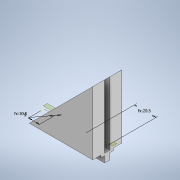
# Autodesk Inventor part: PCB_Mount_Triangle
Saved by Autodesk Inventor 2022 (Build 260153000, 153)
## iProperties
Created: 2024-03-14
Part Number: PCB_Mount_Triangle
Material: Generic
Document SubType Name: Modeling
Designer: Gotham City
Density: 1 g/cm^3
Appearance: Default
Author: Gotham City
Autodesk Inventor part; units mm, degrees
ref_plane "YZ Plane" through (0, 0, 0) normal (1, 0, 0) x (0, 1, 0)
ref_plane "XZ Plane" through (0, 0, 0) normal (0, 1, 0) x (-1, 0, 0)
ref_plane "XY Plane" through (0, 0, 0) normal (0, 0, 1) x (1, 0, 0)
sketch "Sketch1" plane through (0, 0, 0) normal (0, 0, 1) x (1, 0, 0)
  line L0 (0, 60) -> (-60, 0)
  line L1 (-60, 0) -> (0, 0)
  line L2 (0, 0) -> (0, 60)
  dimension "d0" = 45
  dimension "d1" = 60
  constraints: 6 end point, 1 horizontal, 1 perpendicular
  measures "d0" angle of L1 L0
  measures "d1" distance of L1.end L0.start
extrude "Extrusion1" add sketch "Sketch1" along normal mid plane 27.5
sketch "Sketch2" plane through (-60, 0, 13.75) normal (0, -1, 0) x (1, 0, 0)
  line L0 (0, 0) -> (0, -27.5) projected
  line L1 (60, -27.5) -> (60, 0) projected
  line L2 (0, -7.75) -> (60, -7.75)
  line L3 (60, -7.75) -> (60, -19.75)
  line L4 (60, -19.75) -> (0, -19.75)
  line L5 (0, -19.75) -> (0, -7.75)
  line L6 (30, -7.75) -> (30, 0) construction
  line L7 (0, 0) -> (60, 0) construction
  line L8 (0, -27.5) -> (60, -27.5) construction
  line L9 (30, -27.5) -> (30, -19.75) construction
  point P0 (60, -13.75)
  point P1 (0, -19.75)
  dimension "d4" = 12
  constraints: 12 end point, 4 midpoint, 2 parallel, 2 point on line, 1 collinear, 1 horizontal, 1 perpendicular
  measures "d4" distance between parallel lines of L4 L2
extrude "Extrusion2" add sketch "Sketch2" along normal blind 2.2
sketch "Sketch3" plane through (-60, -2.2, 13.75) normal (0, -1, 0) x (1, 0, 0)
  line L0 (0, -7.75) -> (0, -19.75) projected
  line L1 (60, -27.5) -> (60, 0) projected
  line L2 (0, -11.25) -> (60, -11.25)
  line L3 (60, -11.25) -> (60, -16.25)
  line L4 (60, -16.25) -> (0, -16.25)
  line L5 (0, -16.25) -> (0, -11.25)
  line L6 (30, -11.25) -> (30, -7.75) construction
  line L7 (0, -19.75) -> (60, -19.75) construction
  line L8 (30, -19.75) -> (30, -16.25) construction
  line L9 (60, -7.75) -> (0, -7.75) construction
  point P0 (60, -13.75)
  point P1 (0, -16.25)
  dimension "d7" = 5
  constraints: 12 end point, 4 midpoint, 2 parallel, 2 point on line, 1 collinear, 1 horizontal, 1 perpendicular, 1 vertical
  measures "d7" distance between parallel lines of L4 L2
extrude "Extrusion3" add sketch "Sketch3" along normal blind 6
ref_plane "Work Plane2" through (-60, 4.8, 13.75) normal (0, -1, 0) x (1, 0, 0)
sketch "Sketch4" plane through (-60, 4.8, 13.75) normal (0, -1, 0) x (1, 0, 0)
  circle A0 centre (10.5, -13.75) radius 4.5
  circle A1 centre (39.5, -13.75) radius 4.5
  line L0 (10.5, -13.75) -> (0, -13.75) construction
  line L1 (60, -16.25) -> (0, -16.25) construction
  line L2 (39.5, -13.75) -> (10.5, -13.75) construction
  line L3 (60, -11.25) -> (0, -11.25) construction
  line L4 (39.5, -13.75) -> (60, -13.75) construction
  line L5 (0, -11.25) -> (0, -16.25) construction
  dimension "d12" = 9
  dimension "d14" = 10.5
  dimension "d30" = 20.5
  constraints: 6 end point, 2 centre point, 2 parallel, 1 equal radius, 1 horizontal, 1 midpoint
  measures "d12" diameter of A0
  measures "d14" distance from line of L5 L0.start
  measures "d30" distance of L2.start L4.end
hole "Hole1" at (-49.5, 4.8, 0) at (-20.5, 4.8, 0) direction (0, -1, 0) diameter 5.5 end through all start extended yes counterbore diameter 10 counterbore depth 0.1 clearance for "Socket Head Cap Screw ISO 4762" size "M5" standard "ISO"
sketch "Sketch5" plane through (-21.6456, -2.2, -2.5) normal (0, 0, -1) x (-1, 0, 0)
  line L0 (38.3544, 0) -> (-21.6456, 0) projected
  line L1 (23.3544, 0) -> (33.3544, 0)
  line L2 (33.3544, 0) -> (33.3544, -6)
  line L3 (33.3544, -6) -> (23.3544, -6)
  line L4 (23.3544, -6) -> (23.3544, 0)
  line L5 (3.3544, 0) -> (-5.6456, 0)
  line L6 (-5.6456, 0) -> (-5.6456, -6)
  line L7 (-5.6456, -6) -> (3.3544, -6)
  line L8 (3.3544, -6) -> (3.3544, 0)
  line L9 (0, -6) -> (26.7087, -6) construction
  line L10 (-21.6456, 7) -> (38.3544, 7) construction
  line L11 (23.3544, 7) -> (32.3544, 7) projected
  point P0 (33.3544, 7)
  point P1 (42.3544, 7)
  point P2 (-5.6456, 7)
  point P3 (3.3544, 7)
  constraints: 16 end point, 4 parallel, 4 vertical alignment, 3 point on line, 2 horizontal, 2 perpendicular, 1 horizontal alignment
extrude "Extrusion5" cut sketch "Sketch5" along normal through all both and the other way through all
sketch "Sketch6" plane through (0, 0, 13.75) normal (1, 0, 0) x (0, 0, -1)
  line L0 (27.5, 60) -> (0, 60) projected
  line L1 (7.75, 0) -> (0, 0) projected
  line L2 (16.25, 60) -> (11.25, 60)
  line L3 (11.25, 60) -> (11.25, 0)
  line L4 (11.25, 0) -> (16.25, 0)
  line L5 (16.25, 0) -> (16.25, 60)
  line L6 (16.25, 30) -> (27.5, 30) construction
  line L7 (0, 0) -> (0, 60) construction
  line L8 (0, 30) -> (11.25, 30) construction
  line L9 (27.5, 60) -> (27.5, 0) construction
  point P0 (13.75, 0)
  dimension "d27" = 5
  constraints: 12 end point, 4 midpoint, 2 horizontal, 2 parallel, 2 point on line, 1 collinear, 1 perpendicular
  measures "d27" distance between parallel lines of L5 L3
extrude "Extrusion6" cut sketch "Sketch6" against normal blind 10
sketch "Sketch7" plane through (-25, -2.2, -2.5) normal (0, 0, -1) x (-1, 0, 0)
  line L0 (35, -6) -> (30, -6) projected
  line L1 (30, 0) -> (30, -6) projected
  line L2 (35, -6) -> (30, -6)
  line L3 (30, -6) -> (30, 0)
  line L4 (30, 0) -> (35, 0)
  line L5 (35, 0) -> (35, -6)
  line L6 (35, 0) -> (-25, 0) projected
  line L7 (20, 0) -> (14, -6)
  line L8 (20, -6) -> (0, -6) projected
  line L9 (20, -6) -> (20, 0) projected
  line L10 (14, -6) -> (20, -6)
  line L11 (20, -6) -> (20, 0)
  line L12 (-9, 0) -> (-9, -6) projected
  line L13 (-9, -6.0008) -> (-9, 0)
  line L14 (-9, 0) -> (-15, -6)
  line L15 (-25, -6) -> (-9, -6) projected
  line L16 (-15, -6) -> (-9, -6)
  point P0 (-25, 2.2)
  dimension "d40" = 45
  dimension "d41" = 45
  constraints: 20 end point, 4 point on line, 3 horizontal, 2 parallel, 2 perpendicular, 1 collinear
  measures "d40" angle of L9 L7
  measures "d41" angle of L14 L13
extrude "Extrusion7" cut sketch "Sketch7" against normal through all
sketch "Sketch8" plane through (0, 0, 2.5) normal (0, 0, -1) x (-1, 0, 0)
  line L0 (0, 0) -> (0, 60) projected
  line L1 (10, 50) -> (10, 0) projected
  line L2 (0, 20) -> (10, 20)
  line L3 (10, 20) -> (10, 40)
  line L4 (10, 40) -> (0, 40)
  line L5 (0, 40) -> (0, 20)
  line L6 (6, 20) -> (6, 40)
  point P0 (10, 20)
  dimension "d45" = 20
  dimension "d46" = 20
  dimension "d47" = 4
  constraints: 10 end point, 4 point on line, 2 parallel, 2 perpendicular, 1 horizontal
  measures "d45" distance from line of L0.start L2
  measures "d46" distance between parallel lines of L2 L4
  measures "d47" distance between parallel lines of L6 L1
extrude "Extrusion8" add sketch "Sketch8" along normal up to surface (5 mm away) contours L6 L4 L1 L2
chamfer "Chamfer4" distance 4 angle 45 1 edges at (-6, 40, 0)
thicken "Thicken1" operation add thickness 0.1 both sides no extend neighbours yes toward (0, 0, -1) faces at (-2, 32, -2.5)
thicken "Thicken2" operation add thickness 0.1 both sides no extend neighbours yes toward (0, 0, 1) faces at (-2, 32, 2.5)
thicken "Thicken3" operation add thickness 0.1 both sides no extend neighbours yes toward (0, 1, 0) faces at (-8.6667, 20, -0.8667) (-6, 30.6667, 0.8667) (-7.3333, 37.3334, 0.8667)
equation "\"d41\" = d40"
body "Solid1"
